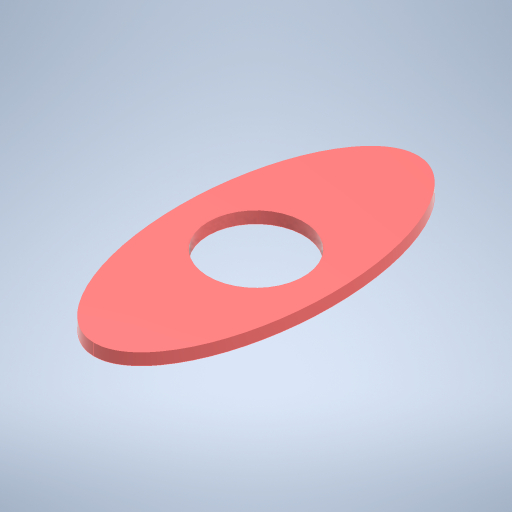
# Autodesk Inventor part: Smoke visualization bottom
Saved by Autodesk Inventor 2023 (Build 270158000, 158)
## iProperties
Created: 2022-09-27
Part Number: Smoke visualization bottom
Material: ABS Plastic
Document SubType Name: Modeling
Designer: earls
Density: 1.06 g/cm^3
Appearance: Smooth - Red
Author: earls
Autodesk Inventor part; units mm, degrees
ref_plane "YZ Plane" through (0, 0, 0) normal (1, 0, 0) x (0, 1, 0)
ref_plane "XZ Plane" through (0, 0, 0) normal (0, 1, 0) x (-1, 0, 0)
ref_plane "XY Plane" through (0, 0, 0) normal (0, 0, 1) x (1, 0, 0)
sketch "Sketch1" plane through (0, 0, 0) normal (0, 1, 0) x (-1, 0, 0)
  spline S0 degree 3 poles (0, 34) (0.3248, 34) (0.9745, 33.9562) (1.7877, 33.791) (2.6017, 33.5418) (3.2534, 33.2745) (4.0665, 32.8541) (4.715, 32.4483) (5.6805, 31.7352) (6.6338, 30.8829) (7.8695, 29.5199) (8.7621, 28.3323) (9.6192, 27.0199) (10.1717, 26.0841) (10.9682, 24.5938) (11.7196, 22.9912) (12.7508, 20.3975) (13.5577, 17.9049) (14.414, 14.5976) (14.9722, 11.8163) (15.5011, 8.2166) (15.7862, 5.2578) (15.965, 1.5094) (15.965, -1.5094) (15.7862, -5.2578) (15.5011, -8.2166) (14.9722, -11.8163) (14.414, -14.5976) (13.5577, -17.9049) (12.7508, -20.3975) (11.7196, -22.9912) (10.9682, -24.5938) (10.1717, -26.0841) (9.6192, -27.0199) (8.7621, -28.3323) (7.8695, -29.5199) (6.6338, -30.8829) (5.6805, -31.7352) (4.715, -32.4483) (4.0665, -32.8541) (3.2534, -33.2745) (2.6017, -33.5418) (1.7877, -33.791) (1.1371, -33.9231) (0.3248, -34.0055) (-0.3248, -34.0055) (-1.1371, -33.9231) (-1.7877, -33.791) (-2.6017, -33.5418) (-3.2534, -33.2745) (-4.0665, -32.8541) (-4.715, -32.4483) (-5.6805, -31.7352) (-6.6338, -30.8829) (-7.8695, -29.5199) (-8.7621, -28.3323) (-9.6192, -27.0199) (-10.1717, -26.0841) (-10.9682, -24.5938) (-11.7196, -22.9912) (-12.7508, -20.3975) (-13.5577, -17.9049) (-14.414, -14.5976) (-14.9722, -11.8163) (-15.5011, -8.2166) (-15.7862, -5.2578) (-15.965, -1.5094) (-15.965, 1.5094) (-15.7862, 5.2578) (-15.5011, 8.2166) (-14.9722, 11.8163) (-14.414, 14.5976) (-13.5577, 17.9049) (-12.7508, 20.3975) (-11.7196, 22.9912) (-10.9682, 24.5938) (-10.1717, 26.0841) (-9.6192, 27.0199) (-8.7621, 28.3323) (-7.8695, 29.5199) (-6.6338, 30.8829) (-5.6805, 31.7352) (-4.715, 32.4483) (-4.0665, 32.8541) (-3.2534, 33.2745) (-2.6017, 33.5418) (-1.7877, 33.791) (-0.9745, 33.9562) (-0.3248, 34) (0, 34) knots -6.283185 -6.283185 -6.283185 -6.283185 -6.217735 -6.152286 -6.119561 -6.054111 -6.021386 -5.955936 -5.923211 -5.825036 -5.759587 -5.661412 -5.628687 -5.563237 -5.530512 -5.432337 -5.366887 -5.235988 -5.170538 -5.039638 -4.974188 -4.843289 -4.777839 -4.646939 -4.581489 -4.45059 -4.38514 -4.25424 -4.18879 -4.057891 -3.992441 -3.894266 -3.861541 -3.796091 -3.763366 -3.665191 -3.599742 -3.501567 -3.468842 -3.403392 -3.370667 -3.305217 -3.272492 -3.207043 -3.174318 -3.108868 -3.076143 -3.010693 -2.977968 -2.912518 -2.879793 -2.814343 -2.781618 -2.683444 -2.617994 -2.519819 -2.487094 -2.421644 -2.388919 -2.290745 -2.225295 -2.094395 -2.028945 -1.898046 -1.832596 -1.701696 -1.636246 -1.505346 -1.439897 -1.308997 -1.243547 -1.112647 -1.047198 -0.916298 -0.850848 -0.752673 -0.719948 -0.654498 -0.621774 -0.523599 -0.458149 -0.359974 -0.327249 -0.261799 -0.229074 -0.163625 -0.1309 -0.06545 0 0 0 0
  spline S1 degree 3 poles (-6.2687, -29.0438) (-5.4863, -29.9281) (-4.5881, -30.7526) (-2.8429, -31.8441) (-2.034, -32.2023) (-0.4086, -32.5372) (0.357, -32.5398) (2.0846, -32.2012) (2.98, -31.7835) (5.0621, -30.4075) (6.3081, -29.1549) (9.3194, -24.942) (10.9197, -21.4805) (13.9972, -10.9319) (14.7722, -3.3794) (13.9609, 10.4109) (12.7309, 16.3149) (9.6608, 24.1376) (8.2643, 26.6053) (5.7386, 29.7244) (4.6873, 30.6823) (2.885, 31.8233) (2.0736, 32.1886) (0.4474, 32.5339) (-0.3168, 32.5422) (-2.0381, 32.217) (-2.929, 31.8093) (-5.0005, 30.4599) (-6.2391, 29.2302) (-9.2337, 25.0936) (-10.8309, 21.6925) (-14.2509, 10.2227) (-14.9756, 1.302) (-13.4611, -13.0289) (-12.1167, -18.3244) (-9.0566, -25.252) (-7.7054, -27.4199) (-6.2687, -29.0438) knots -10.998443 -10.998443 -10.998443 -10.998443 -10.644227 -10.644227 -10.379339 -10.379339 -10.14068 -10.14068 -9.84002 -9.84002 -9.367947 -9.367947 -8.623315 -8.623315 -7.462487 -7.462487 -6.475292 -6.475292 -5.855476 -5.855476 -5.434797 -5.434797 -5.136307 -5.136307 -4.869323 -4.869323 -4.534774 -4.534774 -4.011245 -4.011245 -3.187105 -3.187105 -1.682564 -1.682564 -0.650457 -0.650457 0 0 0 0
  circle A0 centre (0, 0) radius 10
  dimension "d0" = 20
  constraints: 1 centre point, 1 coincident, 2 other
  measures "d0" diameter of A0
extrude "Extrusion1" add sketch "Sketch1" along normal blind 2.5 contours S0 | S1
body "Solid1"
